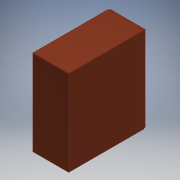
# Autodesk Inventor part: NP18-12 Battery
Saved by Autodesk Inventor 2018 (Build 220112000, 112)
## iProperties
Created: 2017-10-31
Part Number: NP18-12 Battery
Material: Copper
Document SubType Name: Modeling
Designer: P136265
Density: 8.94 g/cm^3
Appearance: Copper - Satin
Author: P136265
Autodesk Inventor part; units mm, degrees
ref_plane "YZ Plane" through (0, 0, 0) normal (1, 0, 0) x (0, 1, 0)
ref_plane "XZ Plane" through (0, 0, 0) normal (0, 1, 0) x (-1, 0, 0)
ref_plane "XY Plane" through (0, 0, 0) normal (0, 0, 1) x (1, 0, 0)
sketch "Sketch1" plane through (0, 0, 0) normal (0, 1, 0) x (-1, 0, 0)
  line L0 (-38, 90) -> (38, 90)
  line L1 (38, 90) -> (38, -90)
  line L2 (38, -90) -> (-38, -90)
  line L3 (-38, -90) -> (-38, 90)
  line L4 (-38, 90) -> (38, -90) construction
  line L5 (38, 90) -> (-38, -90) construction
  point P0 (0, 0)
  dimension "d0" = 76
  dimension "d1" = 180
  constraints: 12 end point, 2 midpoint, 2 parallel, 1 horizontal, 1 perpendicular
  measures "d0" distance of L1.end L2.end
  measures "d1" distance of L0.end L1.end
extrude "Extrusion1" add sketch "Sketch1" along normal blind 162
sketch "Sketch2" plane through (0, 162, 0) normal (0, 1, 0) x (1, 0, 0)
  line L0 (-38, -90) -> (38, -90) construction
  line L1 (38, -90) -> (38, 90) construction
  line L2 (38, 90) -> (-38, 90) construction
  line L3 (-38, 90) -> (-38, -90) construction
  line L4 (-37, -89) -> (37, -89)
  line L5 (37, -89) -> (37, 89)
  line L6 (37, 89) -> (-37, 89)
  line L7 (-37, 89) -> (-37, -89)
  line L8 (-38, 90) -> (-38, -90) projected
  line L9 (-38, -90) -> (38, -90)
  line L10 (38, -90) -> (38, 90)
  line L11 (38, 90) -> (-38, 90)
  line L12 (-38, 90) -> (-38, -90)
  point P0 (0, 0)
  dimension "d4" = 1
  constraints: 16 end point, 2 parallel, 1 horizontal, 1 perpendicular, 3 other
  measures "d4" distance between parallel lines of L3 L7
extrude "Extrusion2" cut sketch "Sketch2" against normal blind 5
fillet "Fillet1" radius 1 16 edges at (38, 78.5, -90) (38, 78.5, 90) (-38, 78.5, -90) (-38, 78.5, 90) (0, 0, 90) (-38, 0, 0) (0, 0, -90) (38, 0, 0) (37, 159.5, -89) (37, 162, 0) (0, 162, -89) (37, 159.5, 89) (-37, 159.5, 89) (0, 162, 89) (-37, 162, 0) (-37, 159.5, -89)
sketch "Sketch3" plane through (0, 162, 0) normal (0, 1, 0) x (1, 0, 0)
  line L0 (37, -88) -> (37, 88) construction
  line L1 (-36, -89) -> (36, -89) construction
  line L2 (-37, 88) -> (-37, -88) construction
  line L3 (-32, -78) -> (-26, -78)
  line L4 (-26, -78) -> (-26, -77)
  line L5 (-26, -77) -> (-32, -77)
  line L6 (-32, -77) -> (-32, -78)
  line L7 (-32, -78) -> (-26, -77) construction
  line L8 (-26, -78) -> (-32, -77) construction
  line L9 (26, -78) -> (32, -78)
  line L10 (32, -78) -> (32, -77)
  line L11 (32, -77) -> (26, -77)
  line L12 (26, -77) -> (26, -78)
  line L13 (26, -78) -> (32, -77) construction
  line L14 (32, -78) -> (26, -77) construction
  point P0 (0, 0)
  point P1 (-29, -77.5)
  point P2 (29, -77.5)
  dimension "d12" = 6
  dimension "d13" = 1
  dimension "d14" = 6
  dimension "d15" = 1
  dimension "d16" = 11
  dimension "d17" = 5
  dimension "d18" = 5
  dimension "d19" = 11
  constraints: 24 end point, 4 midpoint, 4 parallel, 2 horizontal, 2 perpendicular
  measures "d12" distance of L5.end L4.end
  measures "d13" distance of L4.end L3.end
  measures "d14" distance of L11.end L10.end
  measures "d15" distance of L10.end L9.end
  measures "d16" distance between parallel lines of L1 L9
  measures "d17" distance between parallel lines of L0 L10
  measures "d18" distance between parallel lines of L2 L6
  measures "d19" distance between parallel lines of L1 L3
extrude "Extrusion3" add sketch "Sketch3" along normal blind 3
sketch "Sketch4" plane through (32, 162, 77) normal (0, 0, -1) x (-1, 0, 0)
  line L0 (-0.25, 2) -> (6.25, 2)
  line L1 (6.25, 2) -> (6.25, 3)
  line L2 (6.25, 3) -> (-0.25, 3)
  line L3 (-0.25, 3) -> (-0.25, 2)
  line L4 (-0.25, 2) -> (6.25, 3) construction
  line L5 (6.25, 2) -> (-0.25, 3) construction
  line L6 (0, 3) -> (6, 3) construction
  line L7 (57.75, 2) -> (64.25, 2)
  line L8 (64.25, 2) -> (64.25, 3)
  line L9 (64.25, 3) -> (57.75, 3)
  line L10 (57.75, 3) -> (57.75, 2)
  line L11 (57.75, 2) -> (64.25, 3) construction
  line L12 (64.25, 2) -> (57.75, 3) construction
  line L13 (58, 3) -> (64, 3) construction
  point P0 (32, -162)
  point P1 (3, 2.5)
  point P2 (3, 3)
  point P3 (61, 2.5)
  point P4 (61, 3)
  dimension "d22" = 6.5
  dimension "d23" = 1
  dimension "d24" = 6.5
  dimension "d25" = 1
  constraints: 24 end point, 8 midpoint, 4 parallel, 2 horizontal, 2 perpendicular
  measures "d22" distance of L2.end L1.end
  measures "d23" distance of L1.end L0.end
  measures "d24" distance of L9.end L8.end
  measures "d25" distance of L8.end L7.end
extrude "Extrusion4" add sketch "Sketch4" along normal blind 10
fillet "Fillet2" radius 0.25 28 edges at (32.25, 164.5, 67) (25.75, 164.5, 67) (32.25, 164.5, 77) (25.75, 164.5, 77) (-25.75, 164.5, 67) (-25.75, 164.5, 77) (-32.25, 164.5, 67) (-32.25, 164.5, 77) (-32.25, 165, 72) (-32.25, 164, 72) (-29, 165, 67) (-29, 164, 67) (-25.75, 164, 72) (-25.75, 165, 72) (-26, 163, 77) (-26, 163.5, 78) (-32, 163, 77) (-32, 163.5, 78) (32.25, 165, 72) (32.25, 164, 72) (32, 163, 77) (32, 163.5, 78) (29, 165, 67) (29, 164, 67) (25.75, 165, 72) (25.75, 164, 72) (26, 163, 77) (26, 163.5, 78)
fillet "Fillet2" radius 1 2 edges at (29, 165, 78) (-29, 165, 78)
body "Solid1"
